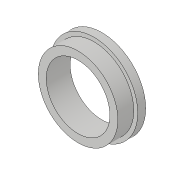
# Autodesk Inventor part: Needle Bearing Stopper
Saved by Autodesk Inventor 2018.3 (Build 223284000, 284)
## iProperties
Created: 2019-04-12
Part Number: Needle Bearing Stopper
Material: Generic
Document SubType Name: Modeling
Designer: aye06091
Mass: 0.405341 g
Surface Area: 6.61095 cm^2
Volume: 0.405341 cm^3
Density: 1 g/cm^3
Appearance: Default
Author: aye06091
Autodesk Inventor part; units mm, degrees
ref_plane "YZ Plane" through (0, 0, 0) normal (1, 0, 0) x (0, 1, 0)
ref_plane "XZ Plane" through (0, 0, 0) normal (0, 1, 0) x (-1, 0, 0)
ref_plane "XY Plane" through (0, 0, 0) normal (0, 0, 1) x (1, 0, 0)
sketch "Sketch1" plane through (0, 0, 0) normal (0, 0, 1) x (1, 0, 0)
  circle A0 centre (0, 0) radius 6.35
  circle A1 centre (0, 0) radius 8.7313
  circle A2 centre (0, 0) radius 7.9375
  dimension "d0" = 12.7
  dimension "d3" = 17.4625
  dimension "d4" = 0.7937
  constraints: 3 centre point, 3 coincident
  measures "d0" diameter of A0
  measures "d3" diameter of A1
  measures "d4" radial gap between concentric circles of A1 A2
extrude "Extrusion1" add sketch "Sketch1" along normal blind 1.5875 contours A0 | A1 | A2
sketch "Sketch2" plane through (0, 0, 1.5875) normal (0, 0, 1) x (1, 0, 0)
  circle A0 centre (0, 0) radius 6.35
  circle A1 centre (0, 0) radius 8.7313
  circle A2 centre (0, 0) radius 7.9375
  dimension "d7" = 12.7
  dimension "d8" = 17.4625
  dimension "d9" = 0.7937
  constraints: 3 centre point, 3 coincident
  measures "d7" diameter of A0
  measures "d8" diameter of A1
  measures "d9" radial gap between concentric circles of A1 A2
extrude "Extrusion2" add sketch "Sketch2" along normal blind 3.175 contours A2
sketch "Sketch3" plane through (0, 0, 1.5875) normal (0, 0, 1) x (1, 0, 0)
  circle A0 centre (0, 0) radius 6.35 projected
  circle A1 centre (0, 0) radius 6.35
  constraints: 1 centre point, 1 coincident, 1 concentric
extrude "Extrusion3" cut sketch "Sketch3" against normal blind 3.175
body "Solid1"
